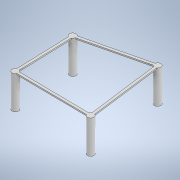
# Autodesk Inventor part: Bauteil125
Saved by Autodesk Inventor 2021 (Build 250183000, 183)
## iProperties
Created: 2021-03-22
Part Number: Bauteil125
Material: Generisch
Document SubType Name: Modeling
Designer: User
Density: 1 g/cm^3
Appearance: Vorgabe
Author: User
Autodesk Inventor part; units mm, degrees
ref_plane "YZ Plane" through (0, 0, 0) normal (1, 0, 0) x (0, 1, 0)
ref_plane "XZ Plane" through (0, 0, 0) normal (0, 1, 0) x (-1, 0, 0)
sketch "Skizze1" plane through (0, 0, 0) normal (0, 1, 0) x (-1, 0, 0)
  line L0 (0, 0) -> (455.0791, 0) construction
  line L1 (455.0791, 0) -> (455.0791, -341.3093) construction
  line L2 (455.0791, -341.3093) -> (0, -341.3093) construction
  line L3 (0, -341.3093) -> (0, 0) construction
  circle A0 centre (842.6138, -408.4047) radius 7.2727
  circle A1 centre (621.1654, -406.0524) radius 7.2727
  line L4 (842.6138, -408.4047) -> (621.1654, -406.0524)
  circle A2 centre (200.2453, -130.8679) radius 2.25 construction
  line L5 (0, 0) -> (200.2453, -130.8679) construction
  circle A3 centre (209.4874, -203.0699) radius 2.25 construction
  line L6 (0, 0) -> (209.4874, -203.0699) construction
  circle A4 centre (273.7033, -187.514) radius 2.25 construction
  circle A5 centre (271.829, -131.6232) radius 2.25 construction
  line L7 (0, 0) -> (271.829, -131.6232) construction
  line L8 (273.7033, -187.514) -> (0, 0) construction
  circle A6 centre (273.7033, -187.514) radius 3.4 construction
  circle A7 centre (273.7033, -187.514) radius 4.4 construction
  line L9 (264.5116, -185.8873) -> (267.409, -191.0479) construction
  arc A8 (267.409, -191.0479) -> (279.9975, -183.9801) centre (273.7033, -187.514) ccw construction
  line L10 (279.9975, -183.9801) -> (277.2184, -179.0301) construction
  line L11 (277.2372, -193.8083) -> (273.7033, -187.514) construction
  line L12 (276.2794, -191.081) -> (277.6647, -193.5484) construction
  line L13 (275.4074, -191.5706) -> (276.7927, -194.0379) construction
  line L14 (273.7033, -187.514) -> (279.9975, -183.9801) construction
  line L15 (273.7033, -187.514) -> (267.409, -191.0479) construction
  line L16 (273.7033, -187.514) -> (270.1693, -181.2197) construction
  line L17 (289.1642, -172.2158) -> (260.8104, -188.135) construction
  line L18 (277.2703, -184.9379) -> (279.7528, -183.5441) construction
  line L19 (277.7598, -185.8098) -> (280.2272, -184.4245) construction
  line L20 (271.9991, -183.4574) -> (271.3143, -182.2376) construction
  line L21 (271.1271, -183.947) -> (270.4423, -182.7272) construction
  line L22 (270.1362, -190.0901) -> (267.6689, -191.4754) construction
  line L23 (269.6467, -189.2181) -> (267.1642, -190.6119) construction
  circle A9 centre (273.7033, -187.514) radius 3
  circle A10 centre (273.7033, -187.514) radius 1.7711
  circle A11 centre (209.4874, -203.0699) radius 3
  circle A12 centre (209.4874, -203.0699) radius 1.7711
  circle A13 centre (200.2453, -130.8679) radius 3
  circle A14 centre (200.2453, -130.8679) radius 1.7711
  circle A15 centre (271.829, -131.6232) radius 3
  circle A16 centre (271.829, -131.6232) radius 1.7711
  line L24 (273.1205, -134.3309) -> (274.8104, -184.7258)
  line L25 (270.7218, -134.4114) -> (272.4118, -184.8062)
  line L26 (271.9295, -134.6215) -> (273.6027, -184.5157) construction
  line L27 (270.7876, -188.2203) -> (212.4031, -202.3636) construction
  line L28 (209.1065, -200.0941) -> (200.6262, -133.8436) construction
  line L29 (203.2451, -130.8995) -> (268.8292, -131.5915) construction
  line L30 (271.3135, -189.3276) -> (212.4422, -203.5888)
  line L31 (211.8771, -201.2563) -> (270.7485, -186.9951)
  line L32 (210.3286, -200.1902) -> (201.7847, -133.4428)
  line L33 (199.4041, -133.7475) -> (207.948, -200.4949)
  line L34 (203.0073, -129.6969) -> (269.0923, -130.3942)
  line L35 (269.0669, -132.7941) -> (202.982, -132.0968)
  dimension "d101" = 8.8
  dimension "d41" = 4.5
  dimension "d46" = 33.166
  dimension "d47" = 4.5
  dimension "d51" = 44.109
  dimension "d68" = 239.2166
  dimension "d73" = 291.7573
  dimension "d74" = 4.5
  dimension "d75" = 4.5
  dimension "d92" = 25.837
  dimension "d93" = 34.415
  dimension "d94" = 302.0193
  dimension "d95" = 331.7755
  dimension "d97" = 341.3093
  dimension "d102" = 1
  dimension "d104" = 14.437
  dimension "d141" = 1
  dimension "d165" = 90
  dimension "d168" = 1
  dimension "d170" = 1
  dimension "d172" = 1
  dimension "d173" = 0.4
  dimension "d174" = 3.5423
  dimension "d175" = 6
  dimension "d176" = 6
  dimension "d177" = 3.5423
  dimension "d178" = 6
  dimension "d179" = 3.5423
  dimension "d180" = 6
  dimension "d181" = 3.5423
  dimension "d185" = 2.4
  dimension "d187" = 2.4
  dimension "d191" = 2.4
  dimension "d192" = 2.4
  dimension "d237" = 55.9222
  constraints: 66 end point, 24 point on circle, 15 centre point, 13 coincident, 10 parallel, 8 line through centre, 4 point on line, 3 collinear, 2 perpendicular, 1 horizontal, 33 other
  measures "d41" diameter of A2
  measures "d46" angle of L5 L0
  measures "d47" diameter of A3
  measures "d51" angle of L6 L0
  measures "d68" distance of L0.start L5.end
  measures "d73" distance of L0.start L6.end
  measures "d74" diameter of A5
  measures "d75" diameter of A4
  measures "d92" angle of L0 L7
  measures "d93" angle of L0 L8
  measures "d94" distance of L0.start L7.end
  measures "d95" distance of L8.start L0.start
  measures "d97" distance of L0.end L1.end
  measures "d104" distance between parallel lines of L9 L10
  measures "d141" distance between parallel lines of L12 L13
  measures "d165" angle of L11 L17
  measures "d168" distance between parallel lines of L19 L18
  measures "d170" distance between parallel lines of L21 L20
  measures "d172" distance between parallel lines of L23 L22
  measures "d173" radial gap between concentric circles of A6 A9
  measures "d174" diameter of A10
  measures "d175" diameter of A9
  measures "d176" diameter of A11
  measures "d177" diameter of A12
  measures "d178" diameter of A13
  measures "d179" diameter of A14
  measures "d180" diameter of A15
  measures "d181" diameter of A16
  measures "d185" distance between parallel lines of L24 L25
  measures "d187" distance between parallel lines of L30 L31
  measures "d191" distance between parallel lines of L35 L34
  measures "d192" distance between parallel lines of L33 L32
  measures "d237" distance of L7.end L8.start
extrude "Extrusion1" add sketch "Skizze1" along normal blind 1.2 contours A9 | A9 L25 A15 L24 | L30 A11 L31 A9 | A15 | A11 | L33 A13 L32 A11 | L35 A13 L34 A15 | A13 | A10 | A12 | A14 | A16
extrude "Extrusion2" add sketch "Skizze1" against normal blind 30 contours A9 | A15 | A11 | A13
sketch "Skizze7" plane through (-271.829, -30, -131.6232) normal (0, -1, 0) x (1, 0, 0)
  circle A0 centre (0, 0) radius 1.7711 projected
  circle A1 centre (71.5837, 0.7553) radius 1.7711 projected
  circle A2 centre (62.3416, -71.4467) radius 1.7711 projected
  circle A3 centre (-1.8743, -55.8908) radius 1.7711 projected
  point P0 (271.829, 131.6232)
  constraints: 4 coincident
ref_plane "Arbeitsebene1" through (-271.829, -30, -131.6232) normal (-0.0105506, 0, 0.9999443) x (0.9999443, 0, 0.0105506)
sketch "Skizze5" plane through (-271.829, -30, -131.6232) normal (-0.0105506, 0, 0.9999443) x (0.9999443, 0, 0.0105506)
  line L0 (-1.7711, -0.525) -> (-2.15, -0.3062)
  line L1 (-2.15, -0.3062) -> (-2.15, -0.2187)
  line L2 (-2.15, -0.2187) -> (-1.7711, 0)
  line L3 (-1.7711, 0) -> (-1.7711, 0.0875)
  line L4 (-1.7711, 0.175) -> (-2.2258, 0.175) construction
  line L5 (-2.2258, 0.175) -> (-2.2258, -0.7) construction
  line L6 (-2.2258, -0.7) -> (-1.7711, -0.7) construction
  line L7 (-1.7711, -0.7) -> (-1.7711, -0.6125) construction
  line L8 (-1.7711, -0.6125) -> (-1.7711, -0.525)
  line L9 (-1.7711, 0.0875) -> (-1.7711, 0.175) construction
  line L10 (-1.7711, -0.525) -> (-1.7711, 0) construction
  line L11 (-2.15, -0.3062) -> (-2.2258, -0.2625) construction
  line L12 (-2.15, -0.2187) -> (-2.2258, -0.2625) construction
  line L13 (0, -0.7) -> (0, 0.175) construction
  line L14 (-1.7711, -0.7) -> (-1.6196, -0.6125) construction
  line L15 (-1.6196, -0.6125) -> (-1.7711, -0.525) construction
  line L16 (-1.7711, 0) -> (-1.6196, 0.0875) construction
  line L17 (-1.6196, 0.0875) -> (-1.7711, 0.175) construction
  line L18 (-1.7711, -0.2625) -> (-2.2258, -0.2625) construction
  line L19 (-1.6196, -0.6125) -> (-1.6196, 0.0875) construction
  line L20 (0, -0.7) -> (-1.7711, -0.7) construction
  line L21 (0, 0.175) -> (-1.7711, 0.175) construction
  line L22 (-3, 0) -> (-3, 31.2) projected
  line L23 (-1.7711, 0) -> (-1.7711, 30) projected
  line L24 (1.7711, 0) -> (-1.7711, 0) projected
  line L25 (-3, 0) -> (3, 0) projected
  line L26 (-1.7711, -0.525) -> (-1.7711, 0)
  dimension "d214" = 60
  dimension "d215" = 4.3
  dimension "d216" = 0.7
  dimension "d217" = 3.5423
  dimension "d218" = 0.3789
  dimension "d219" = 0.0758
  dimension "d226" = 90
  constraints: 46 end point, 11 collinear, 5 parallel, 3 midpoint, 3 perpendicular, 2 coincident, 2 point on line, 9 other
  measures "d214" angle of L0 L2
  measures "d215" diameter of L0.end L13
  measures "d216" distance of L7.end L3.end
  measures "d217" diameter of L7.end L13
  measures "d218" distance between parallel lines of L1 L10
  measures "d219" distance from line of L18.end L1
  measures "d226" angle of L21 L23
coil "Spirale1" sketch "Skizze5" operation cut axis through (-271.829, -30.7, -131.6232) along (0, 1, 0) pitch 0.7 turns 10 hand right
sketch "Skizze8" plane through (-200.2453, -30, -130.8679) normal (0, -1, 0) x (1, 0, 0)
  circle A0 centre (-9.2421, -72.202) radius 1.7711 projected
  circle A1 centre (-73.458, -56.6461) radius 1.7711 projected
  arc A2 (0.8412, -2.8797) -> (-2.7621, 1.1709) centre (0, 0) ccw projected
  point P0 (200.2453, 130.8679)
  constraints: 3 coincident
pattern_sketch "Skizzenbasierte Anordnung1" of "Spirale1" from (-271.829, -30, -131.6232) copies at (-209.4874, -30, -203.0699) at (-273.7033, -30, -187.514) at (-200.2453, -30, -130.8679)
equation "\"d220\" = 60deg"
equation "\"d221\" = 4.3"
equation "\"d222\" = 0.7"
equation "\"d223\" = 3.54225"
equation "\"d224\" = 0.6062"
equation "\"d244\" = 60deg"
equation "\"d245\" = 6.3"
equation "\"d246\" = 1"
equation "\"d247\" = 5.2175"
equation "\"d248\" = 0.866"
